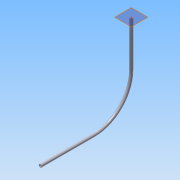
# Autodesk Inventor part: тефлон
Saved by Autodesk Inventor 2017 (Build 210142000, 142)
## iProperties
Part Number: тефлон
Material: Типовые
Document SubType Name: Modeling
Designer: Max
Mass: 1.96544 g
Surface Area: 39.4973 cm^2
Volume: 1.96544 cm^3
Density: 1 g/cm^3
Appearance: Белая холодная
Author: Max
Autodesk Inventor part; units mm, degrees
ref_plane "YZ Plane" through (0, 0, 0) normal (1, 0, 0) x (0, 1, 0)
ref_plane "XZ Plane" through (0, 0, 0) normal (0, 1, 0) x (-1, 0, 0)
ref_plane "XY Plane" through (0, 0, 0) normal (0, 0, 1) x (1, 0, 0)
ref_plane "РабПлоскость2" through (0, 0, -70) normal (0, 0, -1) x (-1, 0, 0)
sketch "Эскиз4" plane through (0, 0, 0) normal (1, 0, 0) x (0, 1, 0)
  line L0 (-2, -70) -> (2, -70)
  line L1 (-50, -180) -> (-120, -180)
  arc A0 (-50, -180) -> (0, -130) centre (-50, -130) ccw
  line L2 (0, -130) -> (0, -70)
  line L3 (2, -70) -> (-250, -70) construction
  dimension "d9" = 60
  dimension "d11" = 50
  dimension "d13" = 70
  constraints: 8 end point, 2 point on circle, 2 tangent, 1 centre point, 1 horizontal, 1 midpoint, 1 perpendicular
  measures "d9" distance of L2.start L2.end
  measures "d11" distance from line of L1 L2.start
  measures "d13" distance of L1.start L1.end
sketch "Эскиз5" plane through (0, 0, -70) normal (0, 0, -1) x (-1, 0, 0)
  circle A0 centre (0, 0) radius 1 projected
  circle A1 centre (0, 0) radius 2 projected
sweep "Сдвиг2" add profiles "Эскиз5" path "Эскиз4" path curves L2 A0 L1
